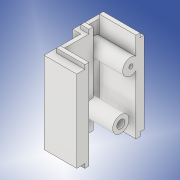
# Autodesk Inventor part: BA003
Saved by Autodesk Inventor 2017 (Build 210142000, 142)
## iProperties
Created: 2017-06-15
Part Number: BA003
Material: ABS Plastic
Document SubType Name: Modeling
Designer: zallen
Density: 1.06 g/cm^3
Appearance: CR White
Author: zallen
Autodesk Inventor part; units mm, degrees
ref_plane "YZ Plane" through (0, 0, 0) normal (1, 0, 0) x (0, 1, 0)
ref_plane "XZ Plane" through (0, 0, 0) normal (0, 1, 0) x (-1, 0, 0)
ref_plane "XY Plane" through (0, 0, 0) normal (0, 0, 1) x (1, 0, 0)
sketch "Sketch1" plane through (0, 0, 0) normal (0, 0, 1) x (1, 0, 0)
  line L0 (0, 0) -> (40, 0)
  line L1 (40, 0) -> (40, 100)
  line L2 (40, 100) -> (0, 100)
  line L3 (0, 100) -> (0, 0)
  dimension "d0" = 40
  dimension "d1" = 100
  constraints: 8 end point, 2 parallel, 1 horizontal, 1 perpendicular
  measures "d0" distance of L2.end L1.end
  measures "d1" distance of L1.end L0.end
extrude "Extrusion1" add sketch "Sketch1" along normal blind 45
sketch "Sketch2" plane through (0, 0, 0) normal (0, 0, -1) x (-1, 0, 0)
  line L0 (-40, 0) -> (-40, 100) projected
  line L1 (-40, 100) -> (10, 100)
  line L2 (10, 100) -> (10, 0)
  line L3 (10, 0) -> (-40, 0)
  line L4 (-40, 0) -> (-40, 100)
  point P0 (0, 0)
  dimension "d4" = 10
  constraints: 8 end point, 2 parallel, 1 horizontal, 1 horizontal alignment, 1 perpendicular
  measures "d4" distance from line of point (0, 0) L2
extrude "Extrusion2" add sketch "Sketch2" along normal blind 37.5
sketch "Sketch3" plane through (40, 0, 45) normal (1, 0, 0) x (0, 0, -1)
  line L0 (82.5, 100) -> (0, 100) projected
  line L1 (0, 0) -> (0, 100) projected
  line L2 (82.5, 0) -> (0, 0) projected
  line L3 (82.5, 100) -> (82.5, 0) projected
  line L4 (5, 5) -> (5, 95)
  line L5 (5, 95) -> (77.5, 95)
  line L6 (77.5, 95) -> (77.5, 5)
  line L7 (77.5, 5) -> (5, 5)
  point P0 (45, 0)
  dimension "d7" = 5
  constraints: 8 end point, 3 other
  measures "d7" distance between parallel lines of L2 L7
extrude "Extrusion3" cut sketch "Sketch3" against normal blind 35 contours L4 L5 L6 L7
sketch "Sketch4" plane through (5, 0, 45) normal (1, 0, 0) x (0, 0, -1)
  line L0 (45, 100) -> (45, 0) projected
  line L1 (45, 100) -> (82.5, 100) projected
  line L2 (82.5, 0) -> (82.5, 100) projected
  line L3 (45, 0) -> (82.5, 0) projected
  line L4 (50, 5) -> (50, 95)
  line L5 (50, 95) -> (77.5, 95)
  line L6 (77.5, 95) -> (77.5, 5)
  line L7 (77.5, 5) -> (50, 5)
  point P0 (45, 0)
  dimension "d10" = 5
  constraints: 8 end point, 3 other
  measures "d10" distance between parallel lines of L0 L4
extrude "Extrusion4" cut sketch "Sketch4" against normal blind 10 contours L4 L5 L6 L7
sketch "Sketch5" plane through (0, 0, 45) normal (0, -1, 0) x (1, 0, 0)
  line L0 (0, 0) -> (40, 0) projected
  line L1 (0, -45) -> (0, 0) projected
  line L2 (-10, -45) -> (0, -45) projected
  line L3 (-10, -45) -> (-10, -82.5) projected
  line L4 (40, -82.5) -> (-10, -82.5) projected
  line L5 (40, -77.5) -> (-5, -77.5)
  line L6 (-5, -77.5) -> (-5, -50)
  line L7 (-5, -50) -> (5, -50)
  line L8 (5, -50) -> (5, -5)
  line L9 (5, -5) -> (40, -5)
  line L10 (40, -77.5) -> (40, -5)
  line L11 (40, -82.5) -> (40, 0) projected
  dimension "d13" = 5
  constraints: 12 end point, 1 collinear, 4 other
  measures "d13" distance between parallel lines of L4 L5
extrude "Extrusion5" cut sketch "Sketch5" against normal through all contours L10 L5 L6 L7 L8 L9
sketch "Sketch6" plane through (0, 100, 45) normal (0, 1, 0) x (1, 0, 0)
  line L0 (0, 45) -> (0, 0) projected
  line L1 (0, 0) -> (40, 0)
  line L2 (40, 0) -> (40, 10)
  line L3 (40, 10) -> (0, 10)
  line L4 (0, 10) -> (0, 0)
  dimension "d16" = 40
  dimension "d17" = 10
  constraints: 8 end point, 2 parallel, 1 horizontal, 1 perpendicular
  measures "d16" distance of L3.end L2.end
  measures "d17" distance of L2.end L1.end
extrude "Extrusion6" add sketch "Sketch6" against normal blind 100
sketch "Sketch8" plane through (40, 100, 35) normal (0, 0, -1) x (-1, 0, 0)
  line L0 (35, 0) -> (35, -100) projected
  line L1 (0, 0) -> (35, 0) projected
  line L2 (0, 0) -> (0, -100) projected
  line L3 (35, -100) -> (0, -100) projected
  line L4 (35, -105) -> (0, -105)
  line L5 (0, -105) -> (0, 5)
  line L6 (0, 5) -> (35, 5)
  line L7 (35, 5) -> (35, -105)
  point P0 (40, -100)
  dimension "d20" = 5
  dimension "d21" = 5
  constraints: 8 end point, 2 parallel, 1 horizontal, 1 perpendicular, 1 point on line
  measures "d20" distance between parallel lines of L4 L3
  measures "d21" distance between parallel lines of L1 L6
extrude "Extrusion7" add sketch "Sketch8" along normal blind 5
sketch "Sketch10" plane through (5, 0, -5) normal (0, 0, -1) x (-1, 0, 0)
  line L0 (0, 0) -> (0, 100) projected
  line L1 (10, 0) -> (0, 0) projected
  line L2 (10, 0) -> (10, 100) projected
  line L3 (0, 100) -> (10, 100) projected
  line L4 (-35, -5) -> (0, -5) projected
  line L5 (10, 0) -> (0, 0)
  line L6 (0, 0) -> (0, -5)
  line L7 (0, -5) -> (10, -5)
  line L8 (10, -5) -> (10, 0)
  line L9 (0, 105) -> (0, 100) projected
  line L10 (10, 100) -> (0, 100)
  line L11 (0, 100) -> (0, 105)
  line L12 (0, 105) -> (10, 105)
  line L13 (10, 105) -> (10, 100)
  point P0 (5, 0)
  constraints: 16 end point, 4 parallel, 2 horizontal, 2 perpendicular
extrude "Extrusion8" add sketch "Sketch10" along normal blind 5
sketch "Sketch11" plane through (5, 0, 45) normal (1, 0, 0) x (0, 0, -1)
  circle A0 centre (32.5, 75) radius 6
  line L0 (15, 100) -> (50, 100) projected
  line L1 (15, 105) -> (15, -5) projected
  circle A1 centre (66.25, 75) radius 6
  circle A2 centre (32.5, 75) radius 10
  circle A3 centre (66.25, 75) radius 10
  point P0 (45, 0)
  dimension "d26" = 12
  dimension "d27" = 25
  dimension "d28" = 17.5
  dimension "d29" = 12
  dimension "d30" = 33.75
  dimension "d31" = 20
  dimension "d32" = 20
  constraints: 4 centre point, 2 coincident, 1 horizontal alignment
  measures "d26" diameter of A0
  measures "d27" distance from line of L0 A0.centre
  measures "d28" distance from line of L1 A0.centre
  measures "d29" diameter of A1
  measures "d30" distance of A1.centre A0.centre
  measures "d31" diameter of A2
  measures "d32" diameter of A3
extrude "Extrusion9" add sketch "Sketch11" along normal blind 35 contours A3
sketch "Sketch12" plane through (-5, 0, 45) normal (1, 0, 0) x (0, 0, -1)
  circle A0 centre (66.25, 75) radius 10 projected
  circle A1 centre (66.25, 75) radius 6 projected
  point P0 (45, 0)
extrude "Extrusion10" add sketch "Sketch12" along normal blind 10
sketch "Sketch14" plane through (-10, 0, 0) normal (-1, 0, 0) x (0, 0, 1)
  circle A0 centre (-21.25, 75) radius 6 projected
  point P0 (0, 0)
extrude "Extrusion12" cut sketch "Sketch14" against normal through all
sketch "Sketch15" plane through (40, 75, -21.25) normal (1, 0, 0) x (0, 0, -1)
  circle A0 centre (0, 0) radius 2.5
  circle A1 centre (0, 0) radius 6 projected
  point P0 (12.5, -75)
  dimension "d41" = 5
  constraints: 1 centre point, 1 coincident
  measures "d41" diameter of A0
extrude "Extrusion13" add sketch "Sketch15" against normal blind 10
sketch "Sketch20" plane through (-5, 0, 45) normal (1, 0, 0) x (0, 0, -1)
  line L0 (77.5, 105) -> (77.5, 105)
  line L1 (77.5, 105) -> (72.5, 105)
  line L2 (72.5, 105) -> (72.5, -5)
  line L3 (72.5, -5) -> (77.5, -5)
  line L4 (77.5, -5) -> (77.5, 105)
  line L5 (82.5, 100) -> (77.5, 100) projected
  line L6 (77.5, 100) -> (77.5, 0) projected
  point P0 (45, 0)
  point P1 (55, -5)
  dimension "d59" = 5
  dimension "d65" = 5
  constraints: 10 end point, 2 horizontal alignment, 2 parallel, 1 horizontal, 1 midpoint, 1 perpendicular, 1 vertical alignment
  measures "d59" distance of L3.end L2.end
  measures "d65" distance between parallel lines of L1 L5
extrude "Extrusion18" add sketch "Sketch20" along normal blind 45
sketch "Sketch22" plane through (5, 0, 45) normal (1, 0, 0) x (0, 0, -1)
  circle A0 centre (54, 20) radius 10
  circle A1 centre (54, 20) radius 5
  line L0 (15, 105) -> (15, -5) projected
  line L1 (72.5, 0) -> (55, 0) projected
  point P0 (45, 0)
  dimension "d66" = 20
  dimension "d67" = 10
  dimension "d68" = 39
  dimension "d69" = 20
  constraints: 2 centre point, 1 coincident
  measures "d66" diameter of A0
  measures "d67" diameter of A1
  measures "d68" distance from line of A0.centre L0
  measures "d69" distance from line of L1 A0.centre
extrude "Extrusion20" add sketch "Sketch22" along normal blind 35
sketch "Sketch23" plane through (-5, 0, 45) normal (1, 0, 0) x (0, 0, -1)
  circle A0 centre (54, 20) radius 5 projected
  circle A1 centre (54, 20) radius 10 projected
  line L0 (55, 105) -> (55, 29.9499) projected
  line L1 (55, 24.899) -> (55, 15.101) projected
  line L2 (55, 10.0501) -> (55, -5) projected
  line L3 (55, 10.0501) -> (55, 29.9499)
  point P0 (45, 0)
  constraints: 2 end point, 1 collinear
extrude "Extrusion21" add sketch "Sketch23" along normal blind 10 contours A0 L3 A1 picked at (62.1905, 21.186)
sketch "Sketch24" plane through (-5, 0, 45) normal (1, 0, 0) x (0, 0, -1)
  circle A0 centre (54, 20) radius 5 projected
  point P0 (45, 0)
extrude "Extrusion22" cut sketch "Sketch24" along normal blind 10
body "Solid1"
